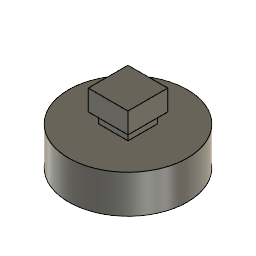
ButtonSpacer (Autodesk Fusion 360 design; units mm, degrees)
Autodesk Fusion 360 part; units mm, degrees
sketch "Sketch1" plane through (0, 0, 0) normal (0, 0, 1) x (1, 0, 0)
  circle A0 centre (0, 0) radius 5.75
  line L0 (1.925, -1.925) -> (-1.925, -1.925)
  line L1 (-1.925, -1.925) -> (-1.925, 1.925)
  line L2 (-1.925, 1.925) -> (1.925, 1.925)
  line L3 (1.925, 1.925) -> (1.925, -1.925)
  line L4 (1.925, -1.925) -> (-1.925, 1.925) construction
  line L5 (-1.925, -1.925) -> (1.925, 1.925) construction
  line L6 (-1.425, 1.425) -> (1.425, 1.425)
  line L7 (1.425, 1.425) -> (1.425, -1.425)
  line L8 (1.425, -1.425) -> (-1.425, -1.425)
  line L9 (-1.425, -1.425) -> (-1.425, 1.425)
  line L10 (-2.05, -2.05) -> (2.05, -2.05)
  line L11 (2.05, -2.05) -> (2.05, 2.05)
  line L12 (2.05, 2.05) -> (-2.05, 2.05)
  line L13 (-2.05, 2.05) -> (-2.05, -2.05)
  line L14 (-2.05, -2.05) -> (2.05, 2.05) construction
  line L15 (2.05, -2.05) -> (-2.05, 2.05) construction
  dimension "d1" = 11.5
  dimension "d2" = 3.85
  dimension "d3" = 3.85
  dimension "d11" = 0.5
  dimension "d12" = 4.1
  dimension "d13" = 4.1
  constraint coincident A0.centre origin
  constraint horizontal L0
  constraint perpendicular L0 L1
  constraint parallel L0 L2
  constraint parallel L1 L3
  constraint coincident L4 A0.centre
  constraint coincident L5 A0.centre
  constraint horizontal L10
  constraint perpendicular L10 L11
  constraint parallel L10 L12
  constraint parallel L11 L13
  constraint coincident L14 A0.centre
  constraint coincident L15 A0.centre
  measures "d1" diameter of A0
  measures "d2" distance of L1.end L2.end
  measures "d3" distance of L0.start L2.end
  measures "d12" distance of L10.start L12.end
  measures "d13" distance of L11.end L12.end
extrude "Extrude1" add sketch "Sketch1" along normal blind 3.7 contours A0 | L0 L1 L2 L3 | L6 L7 L8 L9 | L10 L11 L12 L13
extrude "Extrude2" cut sketch "Sketch1" along normal blind 3.1 contours L0 L1 L2 L3 | L6 L7 L8 L9 | L10 L11 L12 L13
extrude "Extrude3" add sketch "Sketch1" along normal blind 3 from surface at 3.7 contours L0 L1 L2 L3 | L6 L7 L8 L9
extrude "Extrude4" cut sketch "Sketch1" along normal blind 1 from surface at 3.7 contours L0 L1 L2 L3 | L10 L11 L12 L13
